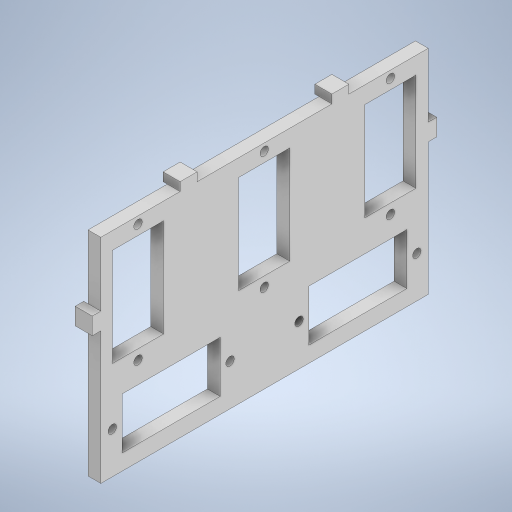
# Autodesk Inventor part: Palm_ServoAttachment
Saved by Autodesk Inventor 2023 (Build 270158000, 158)
## iProperties
Created: 2023-04-20
Part Number: Palm_ServoAttachment
Material: Generic
Document SubType Name: Modeling
Designer: 1senadi
Density: 1 g/cm^3
Appearance: Default
Author: 1senadi
Autodesk Inventor part; units mm, degrees
ref_plane "YZ Plane" through (0, 0, 0) normal (1, 0, 0) x (0, 1, 0)
ref_plane "XZ Plane" through (0, 0, 0) normal (0, 1, 0) x (-1, 0, 0)
ref_plane "XY Plane" through (0, 0, 0) normal (0, 0, 1) x (1, 0, 0)
sketch "Sketch1" plane through (0, 0, 0) normal (1, 0, 0) x (0, 1, 0)
  line L0 (0, 0) -> (0, -76.8)
  line L1 (0, 0) -> (76.8, 0) construction
  line L2 (0, -76.8) -> (-50, -76.8)
  line L3 (-50, -76.8) -> (-50, 0)
  line L4 (-50, 0) -> (0, 0)
  dimension "d0" = 76.8
  dimension "d1" = 90
  dimension "d2" = 50
  constraints: 10 end point, 3 perpendicular, 2 horizontal, 1 vertical
  measures "d0" distance of L0.start L0.end
  measures "d1" angle of L0 L1
  measures "d2" distance of L0.end L2.end
extrude "Extrusion1" add sketch "Sketch1" along normal blind 3
sketch "Sketch2" plane through (0, 0, 0) normal (-1, 0, 0) x (0, 0, 1)
  line L0 (-76.8, -50) -> (-76.8, 0) projected
  line L1 (-76.8, 0) -> (-73.92, 0)
  line L2 (-76.8, 0) -> (0, 0) projected
  line L3 (-73.92, 0) -> (-73.92, -4)
  line L4 (-73.92, -4) -> (-61.92, -4)
  line L5 (-61.92, -4) -> (-61.92, -27)
  line L6 (-61.92, -27) -> (-73.92, -27)
  line L7 (-73.92, -27) -> (-73.92, -4)
  line L8 (-73.92, -4) -> (-38.32, -4)
  line L9 (-38.32, -4) -> (-2.72, -4)
  line L10 (-2.72, -4) -> (-2.72, -27)
  line L11 (-2.72, -27) -> (-14.72, -27)
  line L12 (-14.72, -27) -> (-14.72, -4)
  line L13 (-38.32, -4) -> (-32.32, -4)
  line L14 (-32.32, -4) -> (-32.32, -27)
  line L15 (-32.32, -27) -> (-44.32, -27)
  line L16 (-44.32, -27) -> (-44.32, -4)
  line L17 (-67.92, -27) -> (-67.92, -29.313)
  line L18 (-67.92, -4) -> (-67.92, -1.687)
  circle A0 centre (-67.92, -1.687) radius 1
  circle A1 centre (-67.92, -29.313) radius 1
  line L19 (-38.32, -27) -> (-38.32, -29.313)
  line L20 (-38.32, -4) -> (-38.32, -1.687)
  line L21 (-8.72, -4) -> (-8.72, -1.687)
  line L22 (-8.72, -27) -> (-8.72, -29.313)
  circle A2 centre (-38.32, -1.687) radius 1
  circle A3 centre (-8.72, -1.687) radius 1
  circle A4 centre (-38.32, -29.313) radius 1
  circle A5 centre (-8.72, -29.313) radius 1
  dimension "d5" = 2.88
  dimension "d6" = 4
  dimension "d7" = 12
  dimension "d8" = 23
  dimension "d9" = 12
  dimension "d10" = 35.6
  dimension "d14" = 35.6
  dimension "d15" = 23
  dimension "d16" = 12
  dimension "d17" = 6
  dimension "d18" = 23
  dimension "d19" = 12
  dimension "d24" = 2.313
  dimension "d25" = 2.313
  dimension "d26" = 2
  dimension "d27" = 2
  dimension "d28" = 2
  dimension "d29" = 2
  dimension "d30" = 2
  dimension "d31" = 2
  constraints: 42 end point, 9 perpendicular, 6 centre point, 6 coincident, 6 point on line, 6 vertical, 3 horizontal, 3 midpoint
  measures "d5" distance of L0.end L1.end
  measures "d6" distance of L1.end L3.end
  measures "d7" distance of L3.end L4.end
  measures "d8" distance of L4.end L5.end
  measures "d9" distance of L5.end L6.end
  measures "d10" distance of L3.end L8.end
  measures "d14" distance of L8.end L9.end
  measures "d15" distance of L9.end L10.end
  measures "d16" distance of L10.end L11.end
  measures "d17" distance of L8.end L13.end
  measures "d18" distance of L13.end L14.end
  measures "d19" distance of L14.end L15.end
  measures "d24" distance of L17.start L17.end
  measures "d25" distance of L18.start L18.end
  measures "d26" diameter of A0
  measures "d27" diameter of A1
  measures "d28" diameter of A2
  measures "d29" diameter of A3
  measures "d30" diameter of A4
  measures "d31" diameter of A5
extrude "Extrusion2" cut sketch "Sketch2" against normal up to surface (3 mm away)
sketch "Sketch3" plane through (0, 0, 0) normal (-1, 0, 0) x (0, 0, 1)
  circle A0 centre (-67.92, -29.313) radius 1 projected
  line L0 (-76.8, -50) -> (-76.8, 0) projected
  line L1 (-76.8, -29.313) -> (-76.8, -34.313)
  line L2 (-76.8, -34.313) -> (-71.8, -34.313)
  line L3 (-71.8, -34.313) -> (-48.8, -34.313)
  line L4 (-48.8, -34.313) -> (-48.8, -46.313)
  line L5 (-48.8, -46.313) -> (-71.8, -46.313)
  line L6 (-71.8, -46.313) -> (-71.8, -34.313)
  line L7 (-71.8, -40.313) -> (-74.113, -40.313)
  circle A1 centre (-74.113, -40.313) radius 1
  line L8 (-48.8, -40.313) -> (-46.487, -40.313)
  circle A2 centre (-46.487, -40.313) radius 1
  line L9 (-76.8, 0) -> (0, 0) projected
  line L10 (-38.4, 0) -> (-38.4, -50)
  line L11 (0, -50) -> (-76.8, -50) projected
  line L12 (-5, -34.313) -> (-28, -34.313)
  line L13 (-28, -34.313) -> (-28, -46.313)
  line L14 (-28, -46.313) -> (-5, -46.313)
  line L15 (-5, -46.313) -> (-5, -34.313)
  line L16 (-5, -40.313) -> (-2.687, -40.313)
  circle A3 centre (-2.687, -40.313) radius 1
  line L17 (-28, -40.313) -> (-30.313, -40.313)
  circle A4 centre (-30.313, -40.313) radius 1
  dimension "d32" = 5
  dimension "d33" = 5
  dimension "d34" = 23
  dimension "d35" = 12
  dimension "d36" = 23
  dimension "d37" = 90
  dimension "d38" = 2.313
  dimension "d39" = 2
  dimension "d40" = 2.313
  dimension "d41" = 2
  constraints: 30 end point, 10 symmetric about line, 4 centre point, 4 coincident, 4 midpoint, 3 horizontal, 3 perpendicular, 2 point on line, 2 other
  measures "d32" distance of L1.start L1.end
  measures "d33" distance of L1.end L2.end
  measures "d34" distance of L2.end L3.end
  measures "d35" distance of L3.end L4.end
  measures "d36" distance of L4.end L5.end
  measures "d37" angle of L4 L5
  measures "d38" distance of L7.start L7.end
  measures "d39" diameter of A1
  measures "d40" distance of L8.start L8.end
  measures "d41" diameter of A2
extrude "Extrusion3" cut sketch "Sketch3" against normal up to surface (3 mm away) contours L3 L4 L5 L6 | A1 | A2 | L15 L14 L13 L12 | A3 | A4
sketch "Sketch5" plane through (0, 0, 0) normal (-1, 0, 0) x (0, 0, 1)
  line L0 (-76.8, 0) -> (0, 0) projected
  line L1 (0, 0) -> (-18.6, 0)
  line L2 (0, 0) -> (18.6, 0) construction
  line L3 (-18.6, 0) -> (-22.6, 0)
  line L4 (-22.6, 0) -> (-22.6, 2)
  line L5 (-22.6, 2) -> (-18.6, 2)
  line L6 (-18.6, 2) -> (-18.6, 0)
  line L7 (-38.4, 0) -> (-38.4, -50)
  line L8 (0, -50) -> (-76.8, -50) projected
  line L9 (0, 0) -> (-76.8, 0)
  line L10 (-54.2, 0) -> (-54.2, 2)
  line L11 (-54.2, 2) -> (-58.2, 2)
  line L12 (-58.2, 2) -> (-58.2, 0)
  line L13 (0, 0) -> (0, -15)
  line L14 (0, 0) -> (0, -50) projected
  line L15 (0, -15) -> (0, -19)
  line L16 (0, -19) -> (2, -19)
  line L17 (2, -19) -> (2, -15)
  line L18 (2, -15) -> (0, -15)
  line L19 (-76.8, -15) -> (-76.8, -19)
  line L20 (-76.8, -19) -> (-78.8, -19)
  line L21 (-78.8, -19) -> (-78.8, -15)
  line L22 (-78.8, -15) -> (-76.8, -15)
  point P0 (-58.2, 0)
  dimension "d44" = 18.6
  dimension "d45" = 180
  dimension "d46" = 4
  dimension "d47" = 2
  dimension "d48" = 4
  dimension "d49" = 15
  dimension "d50" = 4
  dimension "d51" = 2
  dimension "d52" = 4
  constraints: 40 end point, 10 symmetric about line, 4 perpendicular, 4 point on line, 2 collinear, 2 midpoint, 1 horizontal
  measures "d44" distance of L0.end L1.end
  measures "d45" angle of L1 L2
  measures "d46" distance of L1.end L3.end
  measures "d47" distance of L3.end L4.end
  measures "d48" distance of L4.end L5.end
  measures "d49" distance of L9.start L13.end
  measures "d50" distance of L13.end L15.end
  measures "d51" distance of L15.end L16.end
  measures "d52" distance of L16.end L17.end
extrude "Extrusion4" add sketch "Sketch5" against normal up to surface (3 mm away) contours L12 L11 L10 L0 | L4 L5 L6 L0 | L14 L18 L17 L16 | L19 L20 L21 L22
sketch "Sketch6" plane through (0, 0, 0) normal (-1, 0, 0) x (0, 0, 1)
  line L0 (-54.2, 2) -> (-58.2, 2) projected
  line L1 (-54.2, 0) -> (-54.2, 2) projected
  line L2 (-58.2, 2) -> (-58.2, 0) projected
  line L3 (-18.6, 2) -> (-22.6, 2) projected
  line L4 (-22.6, 2) -> (-22.6, 0) projected
  line L5 (-18.6, 0) -> (-18.6, 2) projected
  line L6 (2, -15) -> (0, -15) projected
  line L7 (2, -19) -> (2, -15) projected
  line L8 (0, -19) -> (2, -19) projected
  line L9 (-76.8, -15) -> (-78.8, -15) projected
  line L10 (-78.8, -15) -> (-78.8, -19) projected
  line L11 (-78.8, -19) -> (-76.8, -19) projected
  line L12 (-76.8, -15) -> (-76.8, 0) projected
  line L13 (-76.8, -15) -> (-76.8, -19)
  line L14 (-76.8, 0) -> (-58.2, 0) projected
  line L15 (-58.2, 0) -> (-54.2, 0)
  line L16 (-54.2, 0) -> (-22.6, 0) projected
  line L17 (-18.6, 0) -> (0, 0) projected
  line L18 (-22.6, 0) -> (-18.6, 0)
  line L19 (0, 0) -> (0, -15) projected
  line L20 (0, -19) -> (0, -50) projected
  line L21 (0, -15) -> (0, -19)
  constraints: 8 end point, 3 collinear, 1 vertical
extrude "Extrusion5" add sketch "Sketch6" along normal blind 1
body "Solid1"
